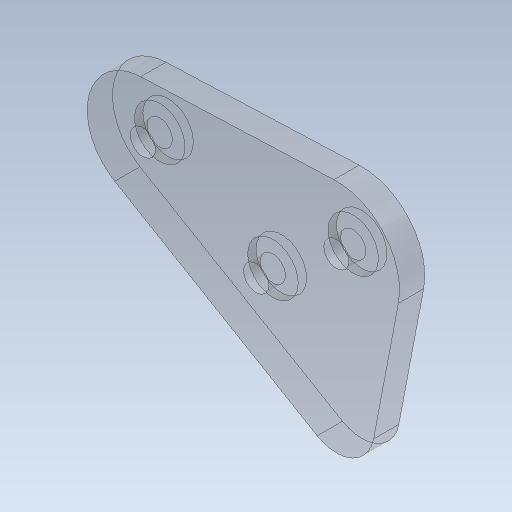
# Autodesk Inventor part: ツイン抑え
Saved by Autodesk Inventor 2020 (Build 240168000, 168)
## iProperties
Created: 2020-01-11
Part Number: ツイン抑え
Material: ポリカーボネート、クリア
Document SubType Name: Modeling
Designer: tanjihayato
Density: 1.2 g/cm^3
Appearance: ポリカーボネート - クリア
Mass: 2.44709 g
Surface Area: 18.3229 cm^2
Volume: 2.03924 cm^3
Author: tanjihayato
Autodesk Inventor part; units mm, degrees
ref_plane "YZ Plane" through (0, 0, 0) normal (1, 0, 0) x (0, 1, 0)
ref_plane "XZ Plane" through (0, 0, 0) normal (0, 1, 0) x (-1, 0, 0)
ref_plane "XY Plane" through (0, 0, 0) normal (0, 0, 1) x (1, 0, 0)
sketch "スケッチ1" plane through (0, 0, 0) normal (0, 0, 1) x (1, 0, 0)
  circle A0 centre (59.9649, 0.0002) radius 1.5
  circle A1 centre (9.9649, 0.0002) radius 2
  circle A2 centre (-5.0351, 0.0002) radius 2
  circle A3 centre (50.4166, -7.2682) radius 1.5
  circle A4 centre (7.9649, -9.9998) radius 1.5
  arc A5 (-5.2274, 4.9965) -> (-7.9614, -4.054) centre (-5.0351, 0.0002) ccw
  line L0 (-7.9614, -4.054) -> (5.3313, -13.6486)
  arc A6 (5.3313, -13.6486) -> (7.4492, -14.4702) centre (7.9649, -9.9998) ccw
  line L1 (7.4492, -14.4702) -> (59.4492, -20.4691)
  arc A7 (59.4492, -20.4691) -> (64.3851, -16.8426) centre (59.9649, -15.9988) ccw
  line L2 (64.3851, -16.8426) -> (67.3319, -1.4061)
  arc A8 (67.3319, -1.4061) -> (59.6765, 7.4946) centre (59.9649, 0.0002) ccw
  line L3 (59.6765, 7.4946) -> (-5.2274, 4.9965)
  circle A9 centre (59.9649, 0.0002) radius 3
  circle A10 centre (50.4166, -7.2682) radius 3
  circle A11 centre (7.9649, -9.9998) radius 3
  circle A12 centre (36.9539, 0.0002) radius 1.5
  circle A13 centre (36.9539, 0.0002) radius 3
  arc A14 (36.6995, 6.6103) -> (33.5984, -5.7005) centre (36.9539, 0.0002) ccw
  line L4 (7.4492, -14.4702) -> (59.4492, -20.4691)
  arc A15 (57.6822, -19.8768) -> (59.4492, -20.4691) centre (59.9649, -15.9988) ccw
  line L5 (33.5984, -5.7005) -> (57.6822, -19.8768)
  line L6 (59.6765, 7.4946) -> (-5.2274, 4.9965)
  point P0 (0, 0)
  point P1 (0, 0)
  dimension "d0" = 6
  dimension "d1" = 6
  dimension "d2" = 6
  dimension "d3" = 6
  constraints: 16 centre point, 14 end point, 12 point on circle, 6 coincident, 3 tangent, 1 point on line
  measures "d0" diameter of A9
  measures "d1" diameter of A10
  measures "d2" diameter of A11
  measures "d3" diameter of A13
extrude "押し出し1" add sketch "スケッチ1" along normal blind 3 contours L3 A8 L2 A7 A15 L5 A14 | A9 | A10 | A13
extrude "押し出し2" cut sketch "スケッチ1" along normal blind 1 contours A9 | A10 | A13
sketch "スケッチ2" plane through (0, 0, 0) normal (0, 0, -1) x (-1, 0, 0)
  circle A0 centre (-59.9649, 0.0002) radius 3 projected
  circle A1 centre (-50.4166, -7.2682) radius 3 projected
  circle A2 centre (-36.9539, 0.0002) radius 3 projected
  line L0 (-59.6765, 7.4946) -> (-36.6995, 6.6103) projected
  arc A3 (-59.6765, 7.4946) -> (-67.3319, -1.4061) centre (-59.9649, 0.0002) ccw projected
  line L1 (-64.3851, -16.8426) -> (-67.3319, -1.4061) projected
  arc A4 (-64.3851, -16.8426) -> (-57.6822, -19.8768) centre (-59.9649, -15.9988) ccw projected
  line L2 (-33.5984, -5.7005) -> (-57.6822, -19.8768) projected
  arc A5 (-33.5984, -5.7005) -> (-36.6995, 6.6103) centre (-36.9539, 0.0002) ccw projected
  circle A6 centre (-59.9649, 0.0002) radius 1.5 projected
  circle A7 centre (-50.4166, -7.2682) radius 1.5 projected
  circle A8 centre (-36.9539, 0.0002) radius 1.5 projected
  point P0 (0, 0)
